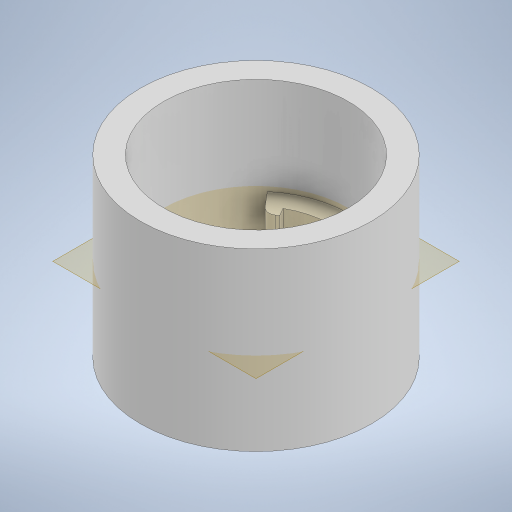
# Autodesk Inventor part: kumi2
Saved by Autodesk Inventor 2023.2 (Build 272271000, 271)
## iProperties
Created: 2022-12-16
Part Number: kumi2
Material: 一般
Document SubType Name: Modeling
Designer: 千葉 俊輔
Density: 1 g/cm^3
Appearance: 既定
Author: 千葉 俊輔
Autodesk Inventor part; units mm, degrees
ref_plane "YZ Plane" through (0, 0, 0) normal (1, 0, 0) x (0, 1, 0)
ref_plane "XZ Plane" through (0, 0, 0) normal (0, 1, 0) x (-1, 0, 0)
ref_plane "XY Plane" through (0, 0, 0) normal (0, 0, 1) x (1, 0, 0)
sketch "スケッチ1" plane through (0, 0, 0) normal (0, 1, 0) x (-1, 0, 0)
  circle A0 centre (0, 0) radius 12.5
  dimension "d0" = 25
  constraints: 1 centre point, 1 coincident
  measures "d0" diameter of A0
extrude "押し出し1" add sketch "スケッチ1" along normal blind 2
sketch "スケッチ2" plane through (0, 2, 0) normal (0, 1, 0) x (1, 0, 0)
  circle A0 centre (0, 0) radius 12.5
  circle A1 centre (0, 0) radius 10
  dimension "d3" = 25
  dimension "d4" = 20
  constraints: 2 centre point, 2 coincident
  measures "d3" diameter of A0
  measures "d4" diameter of A1
extrude "押し出し2" add sketch "スケッチ2" along normal blind 17
sketch "スケッチ3" plane through (0, 2, 0) normal (0, 1, 0) x (1, 0, 0)
  arc A0 (-6.4279, -7.6604) -> (0, -10) centre (0, 0) ccw
  line L0 (0, 0) -> (-6.4279, -7.6604) construction
  line L1 (0, 0) -> (0, -10) construction
  arc A1 (6.4279, 7.6604) -> (0, 10) centre (0, 0) ccw
  line L2 (0, 0) -> (6.4279, 7.6604) construction
  line L3 (0, 0) -> (0, 10) construction
  circle A2 centre (0, 0) radius 10 projected
  line L4 (-6.4279, -7.6604) -> (0, 0)
  line L5 (0, 0) -> (6.4279, 7.6604)
  line L6 (0, -10) -> (0, 0)
  line L7 (0, 10) -> (0, 0)
  circle A3 centre (0, 0) radius 10 projected
  point P0 (3.2139, 3.8302)
  dimension "d8" = 40
  dimension "d10" = 40
  dimension "d11" = 3.8302
  dimension "d12" = 6.4279
  constraints: 16 end point, 4 point on circle, 2 centre point, 2 coincident, 2 collinear, 1 concentric, 1 midpoint
  measures "d8" angle of L0 L1
  measures "d10" angle of L2 L3
  measures "d11" vertical distance of L2.start point (3.214, 3.83)
  measures "d12" horizontal distance of L0.start L0.end
extrude "押し出し3" add sketch "スケッチ3" along normal blind 6.5 contours L4 L6 A0 | A1 L5 L7
sketch "スケッチ4" plane through (0, 8.5, 0) normal (0, 1, 0) x (1, 0, 0)
  line L0 (0, -10) -> (0, 0) projected
  circle A0 centre (0, 0) radius 1
  dimension "d15" = 2
  constraints: 1 centre point, 1 coincident
  measures "d15" diameter of A0
extrude "押し出し4" cut sketch "スケッチ4" against normal blind 7
ref_plane "作業平面1" through (0, 9, 0) normal (0, 1, 0) x (1, 0, 0)
sketch "スケッチ5" plane through (0, 8.5, 0) normal (0, 1, 0) x (1, 0, 0)
  line L0 (0, -10) -> (0, -1) projected
  arc A0 (0, -10) -> (6.4279, -7.6604) centre (0, 0) ccw
  line L1 (0, 0) -> (6.4279, -7.6604) construction
  line L2 (0, 0) -> (0, -10) construction
  arc A1 (0, -8) -> (4, -6.9282) centre (0, 0) ccw
  line L3 (0, 0) -> (4, -6.9282) construction
  line L4 (0, 0) -> (0, -8) construction
  arc A2 (3.5, -6.0622) -> (4.4995, -5.3623) centre (0, 0) ccw
  line L5 (0, 0) -> (4.4995, -5.3623) construction
  line L6 (0, 0) -> (3.5, -6.0622) construction
  arc A3 (0, -10) -> (6.4279, 7.6604) centre (0, 0) ccw projected
  line L7 (0, -10) -> (0, -8)
  line L8 (6.4279, -7.6604) -> (4.4995, -5.3623)
  line L9 (4, -6.9282) -> (3.5, -6.0622)
  line L10 (0, 1) -> (0, 10) projected
  arc A4 (0, 10) -> (-6.4279, 7.6604) centre (0, 0) ccw
  line L11 (0, 0) -> (-6.4279, 7.6604) construction
  line L12 (0, 0) -> (0, 10) construction
  arc A5 (0, 8) -> (-4, 6.9282) centre (0, 0) ccw
  line L13 (0, 0) -> (-4, 6.9282) construction
  line L14 (0, 0) -> (0, 8) construction
  arc A6 (-3.5, 6.0622) -> (-4.4995, 5.3623) centre (0, 0) ccw
  line L15 (0, 0) -> (-3.5, 6.0622) construction
  line L16 (0, 0) -> (-4.4995, 5.3623) construction
  line L17 (-6.4279, 7.6604) -> (-4.4995, 5.3623)
  line L18 (-4, 6.9282) -> (-3.5, 6.0622)
  line L19 (0, 10) -> (0, 8)
  dimension "d19" = 10
  dimension "d20" = 40
  dimension "d21" = 8
  dimension "d22" = 30
  dimension "d23" = 7
  dimension "d24" = 10
  dimension "d25" = 10
  dimension "d26" = 40
  dimension "d27" = 8
  dimension "d28" = 30
  dimension "d29" = 7
  dimension "d30" = 10
  constraints: 36 end point, 12 point on circle, 6 centre point, 6 coincident, 4 collinear, 3 point on line
  measures "d19" radius of A0
  measures "d20" angle of L2 L1
  measures "d21" radius of A1
  measures "d22" angle of L4 L3
  measures "d23" radius of A2
  measures "d24" angle of L6 L5
  measures "d25" radius of A4
  measures "d26" angle of L12 L11
  measures "d27" radius of A5
  measures "d28" angle of L14 L13
  measures "d29" radius of A6
  measures "d30" angle of L15 L16
extrude "押し出し5" add sketch "スケッチ5" against normal blind 5
fillet "フィレット1" radius 1 1 edges at (-4.4995, 6, -5.3623)
fillet "フィレット2" radius 1 1 edges at (4.4995, 6, 5.3623)
